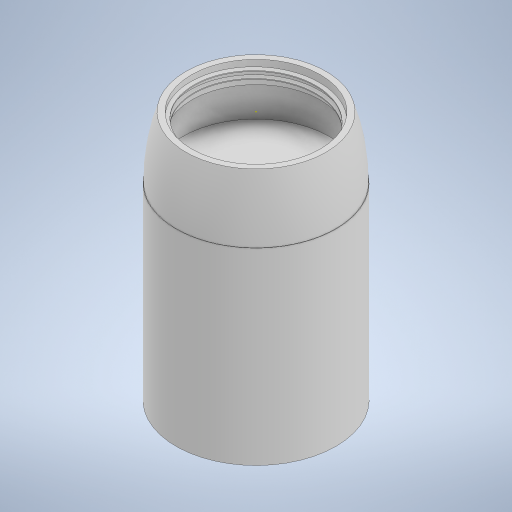
# Autodesk Inventor part: 탄두1
Saved by Autodesk Inventor 2023 (Build 270158000, 158)
## iProperties
Created: 2023-10-03
Part Number: 탄두1
Material: 일반
Document SubType Name: Modeling
Designer: rlatk
Density: 1 g/cm^3
Appearance: 기본값
Author: rlatk
Autodesk Inventor part; units mm, degrees
ref_plane "YZ Plane" through (0, 0, 0) normal (1, 0, 0) x (0, 1, 0)
ref_plane "XZ Plane" through (0, 0, 0) normal (0, 1, 0) x (-1, 0, 0)
ref_plane "XY Plane" through (0, 0, 0) normal (0, 0, 1) x (1, 0, 0)
sketch "스케치1" plane through (0, 0, 0) normal (0, 1, 0) x (-1, 0, 0)
  circle A0 centre (0, 0) radius 46.5
  dimension "d0" = 93
  constraints: 1 centre point, 1 coincident
  measures "d0" diameter of A0
sketch "스케치2" plane through (0, 0, 0) normal (0, 0, 1) x (1, 0, 0)
  line L0 (46.5, 0) -> (-46.5, 0) projected
  line L1 (0, 0) -> (0, 90)
  arc A0 (0, 90) -> (-46.5, 0) centre (59.9038, 2.0372) ccw
  line L2 (-20.2736, 0) -> (-20.2736, 36)
  arc A1 (0, 87.7361) -> (-42.8811, 0) centre (62.0049, 3.084) ccw
  line L3 (0, -19.1775) -> (0, 115.0652) projected
  line L4 (-43.0533, 36) -> (0, 36)
  line L5 (-40.9547, 36) -> (-37.6316, 36)
  line L6 (-37.6316, 36) -> (-37.6316, 23.2038)
  line L7 (-37.6316, 23.2038) -> (-40.9547, 23.2038)
  line L8 (-40.9547, 23.2038) -> (-40.9547, 36)
  point P0 (-43.0533, 28.9768)
  point P1 (-40.9547, 23.3299)
  dimension "d1" = 90
  dimension "d2" = 36
  constraints: 14 end point, 6 point on circle, 4 point on line, 2 centre point, 2 parallel, 2 perpendicular, 1 horizontal, 1 vertical
  measures "d1" distance of L1.start L1.end
  measures "d2" distance of L2.start L2.end
extrude "돌출1" add sketch "스케치1" along normal blind 2
sketch "스케치3" plane through (0, 0, 0) normal (0, -1, 0) x (1, 0, 0)
  circle A0 centre (0, 0) radius 45.75
  circle A1 centre (0, 0) radius 46.7555
  dimension "d6" = 91.5
  constraints: 2 centre point, 2 coincident
  measures "d6" diameter of A0
extrude "돌출2" add sketch "스케치3" along normal blind 110
revolve "회전2" add sketch "스케치2" angle 360 about axis through (0, -10, 0) along (0, 1, 0) contours L0 A0 L8 A1 | L8 L4 A1 | A1 L6 L7 L8
sketch "스케치5" plane through (0, 36, 0) normal (0, 1, 0) x (1, 0, 0)
  point P0 (0, 0)
sketch "스케치6" plane through (0, 0, 0) normal (1, 0, 0) x (0, 1, 0)
  line L0 (36, -37.6316) -> (36, 37.6316) projected
  line L1 (23.2038, -37.6316) -> (23.2038, 37.6316) projected
  line L2 (36, 37.6316) -> (23.2038, 37.6316) projected
  line L3 (23.2038, -37.6316) -> (23.2038, 37.6316) projected
  line L4 (25.7038, 37.6316) -> (24.2038, 37.6316)
  line L5 (24.2038, 37.6316) -> (24.2038, 35.6316)
  line L6 (24.2038, 35.6316) -> (25.7038, 35.6316)
  line L7 (25.7038, 35.6316) -> (25.7038, 37.6316)
  line L8 (25.7038, 37.6316) -> (25.2038, 35.6316)
  line L9 (24.7038, 35.6316) -> (24.2038, 37.6316)
  point P0 (0, 0)
  dimension "d23" = 1.5
  dimension "d24" = 2
  dimension "d25" = 0.5
  dimension "d26" = 0.5
  dimension "d27" = 1
  constraints: 12 end point, 3 point on line, 2 parallel, 1 horizontal, 1 perpendicular
  measures "d23" distance of L6.end L5.end
  measures "d24" distance of L5.end L4.end
  measures "d25" distance of L8.end L6.end
  measures "d26" distance of L5.end L9.start
  measures "d27" distance between parallel lines of L1 L5
coil "코일2" sketch "스케치6" operation add axis through (0, -10, 0) along (0, 1, 0) pitch 4 turns 2 hand right contours L8 L6 L9 L2
